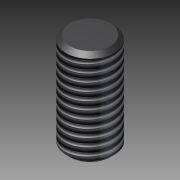
# Autodesk Inventor part: 6mm SHCS
Saved by Autodesk Inventor 2011 (Build 150229000, 229)
## iProperties
Shininess: 64.0
Angle Display Precision: 2
Document Length Units: 11269
Document Angle Units: 11279
Document Time Units: 11290
Document Mass Units: 11283
Document Length Units Precision: 3
Document Angle Units Precision: 2
Compacted: True
Created: 2002-07-24
Part Number: 6mm SHCS
Description: 6mm SHCS
Document SubType Name: Modeling
Designer: PN
Density: 1 g/cm^3
Density: 0.0
Volumn: 0.0
Area: 0.0
PropertySet Name: Model Information
Control State: 0
Master: False
Checked Out: False
Author: PN
Autodesk Inventor part; units mm, degrees
ref_plane "YZ Plane" through (0, 0, 0) normal (1, 0, 0) x (0, 1, 0)
ref_plane "XZ Plane" through (0, 0, 0) normal (0, 1, 0) x (-1, 0, 0)
ref_plane "XY Plane" through (0, 0, 0) normal (0, 0, 1) x (1, 0, 0)
sketch "Sketch1" plane through (0, 0, 0) normal (0, 0, 1) x (1, 0, 0)
  circle A0 centre (0, 0) radius 3
  dimension "d0" = 6
  constraints: 1 centre point, 1 coincident
  measures "d0" diameter of A0
extrude "Extrusion1" add sketch "Sketch1" along normal mid plane 12
chamfer "Chamfer1" distance 0.5 angle 45 2 edges at (-3, 0, 6) (-3, 0, -6)
sketch "Sketch2" plane through (0, 0, -6) normal (0, 0, -1) x (-1, 0, 0)
  circle A0 centre (0, 0) radius 2.5 projected
  line L0 (-1.866, 0) -> (-1, -1.5)
  line L1 (-1, 1.5) -> (-1.866, 0)
  line L2 (1, 1.5) -> (-1, 1.5)
  line L3 (1.866, 0) -> (1, 1.5)
  line L4 (1, -1.5) -> (1.866, 0)
  line L5 (-1, -1.5) -> (1, -1.5)
  circle A1 centre (0, 0) radius 1.616 construction
  dimension "d5" = 3.2321
  dimension "d10" = 1.5
  dimension "d11" = 120
  dimension "d13" = 120
  dimension "d16" = 3
  constraints: 12 end point, 4 tangent, 3 parallel, 1 centre point, 1 coincident, 1 horizontal
  measures "d5" diameter of A1
  measures "d10" distance from line of A0.centre L2
  measures "d11" angle of L5 L0
  measures "d13" angle of L5 L4
  measures "d16" distance between parallel lines of L5 L2
extrude "Extrusion2" cut sketch "Sketch2" against normal blind 4 contours L1 L2 L3 L4 L5 L0
thread "Thread1" size "M6x1" class "6g" standard "ANSI Metric M Profile" full length
body "Solid1"
